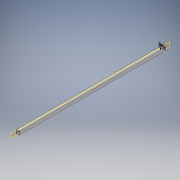
# Autodesk Inventor part: 50x50x5
Saved by Autodesk Inventor 2019 (Build 230136000, 136)
## iProperties
Created: 2022-08-26
Part Number: 50x50x5
Material: Generic
Document SubType Name: Modeling
Designer: laca
Density: 1 g/cm^3
Appearance: Default
Author: laca
Autodesk Inventor part; units mm, degrees
ref_plane "YZ Plane" through (0, 0, 0) normal (1, 0, 0) x (0, 1, 0)
ref_plane "XZ Plane" through (0, 0, 0) normal (0, 1, 0) x (-1, 0, 0)
ref_plane "XY Plane" through (0, 0, 0) normal (0, 0, 1) x (1, 0, 0)
sketch "Sketch1" plane through (0, 0, 0) normal (0, 0, 1) x (1, 0, 0)
  line L0 (-8, 0) -> (-42, 0)
  line L1 (-50, 8) -> (-50, 42)
  line L2 (-42, 50) -> (-8, 50)
  line L3 (0, 42) -> (0, 8)
  arc A0 (-42, 50) -> (-50, 42) centre (-42, 42) ccw
  arc A1 (0, 42) -> (-8, 50) centre (-8, 42) ccw
  arc A2 (-8, 0) -> (0, 8) centre (-8, 8) ccw
  arc A3 (-50, 8) -> (-42, 0) centre (-42, 8) ccw
  line L4 (-45, 42) -> (-45, 8)
  arc A4 (-45, 8) -> (-42, 5) centre (-42, 8) ccw
  line L5 (-42, 5) -> (-8, 5)
  arc A5 (-8, 5) -> (-5, 8) centre (-8, 8) ccw
  line L6 (-5, 8) -> (-5, 42)
  arc A6 (-5, 42) -> (-8, 45) centre (-8, 42) ccw
  line L7 (-8, 45) -> (-42, 45)
  arc A7 (-42, 45) -> (-45, 42) centre (-42, 42) ccw
  point P0 (0, 0)
  point P1 (-50, 50)
  point P2 (-50, 0)
  point P3 (0, 50)
  dimension "d0" = 50
  dimension "d1" = 50
  dimension "d2" = 8
  dimension "d3" = 5
  constraints: 16 end point, 16 point on circle, 8 centre point, 8 point on line, 8 tangent, 4 parallel, 3 equal radius, 2 perpendicular, 1 horizontal, 7 other
  measures "d0" distance of point (-50, 50) point (0, 50)
  measures "d1" distance of point (-50, 0) point (-50, 50)
  measures "d2" radius of A0
  measures "d3" radial gap between concentric circles of A0 A7
extrude "Extrusion1" add sketch "Sketch1" along normal blind 2000
sketch "Sketch2" plane through (-42, 50, 0) normal (0, 1, 0) x (1, 0, 0)
  line L0 (0, 0) -> (34, 0) projected
  line L1 (34, 0) -> (34, -54.5049)
  line L2 (34, 0) -> (34, -2000) projected
  circle A0 centre (12, -100) radius 3
  point P0 (42, 0)
  point P1 (12, -550)
  point P2 (12, -1000)
  point P3 (12, -1450)
  dimension "d6" = 30
  dimension "d7" = 100
  dimension "d10" = 450
  dimension "d22" = 6
  constraints: 2 end point, 1 centre point, 1 coincident, 1 point on line, 1 vertical, 3 other
  measures "d6" horizontal distance of point (42, 0) point (12, -100)
  measures "d7" distance from line of L0 point (12, -100)
  measures "d10" distance of point (12, -100) point (12, -550)
  measures "d22" diameter of A0
extrude "Extrusion2" cut sketch "Sketch2" against normal through all
pattern_linear "Rectangular Pattern1" count 2 spacing 450 along (0, 0, 1) of "Extrusion2"
ref_plane "Work Plane1" through (-30, 50, 550) normal (1, 0, 0) x (0, -1, 0)
body "Solid1"
